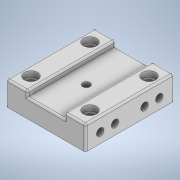
# Autodesk Inventor part: slidescentermount
Saved by Autodesk Inventor 2020 (Build 240168000, 168)
## iProperties
Created: 2019-12-20
Part Number: slidescentermount
Material: Generic
Document SubType Name: Modeling
Designer: xj82b
Density: 1 g/cm^3
Appearance: Default
Author: xj82b
Autodesk Inventor part; units mm, degrees
ref_plane "YZ Plane" through (0, 0, 0) normal (1, 0, 0) x (0, 1, 0)
ref_plane "XZ Plane" through (0, 0, 0) normal (0, 1, 0) x (-1, 0, 0)
ref_plane "XY Plane" through (0, 0, 0) normal (0, 0, 1) x (1, 0, 0)
sketch "Sketch1" plane through (0, 0, 0) normal (0, 1, 0) x (-1, 0, 0)
  line L0 (0, 0) -> (-43, 0)
  line L1 (-43, 0) -> (-43, -48)
  line L2 (-43, -48) -> (0, -48)
  line L3 (0, -48) -> (0, 0)
  circle A0 centre (-21.5, -22) radius 2
  point P0 (-43, -24)
  point P1 (-21.5, -48)
  dimension "d0" = 43
  dimension "d1" = 48
  dimension "d2" = 4
  dimension "d23" = 22
  constraints: 8 end point, 2 midpoint, 2 parallel, 1 centre point, 1 horizontal, 1 perpendicular, 1 vertical alignment
  measures "d0" distance of L2.end L1.end
  measures "d1" distance of L1.end L0.end
  measures "d2" diameter of A0
  measures "d23" distance from line of L0 A0.centre
extrude "Extrusion1" add sketch "Sketch1" along normal blind 13
sketch "Sketch2" plane through (0, 13, 0) normal (0, 1, 0) x (1, 0, 0)
  line L0 (11.5, 54.8346) -> (31.5, 54.8346)
  line L1 (31.5, 54.8346) -> (31.5, -5.4848)
  line L2 (31.5, -5.4848) -> (11.5, -5.4848)
  line L3 (11.5, -5.4848) -> (11.5, 54.8346)
  line L4 (43, 48) -> (0, 48) projected
  point P0 (0, 0)
  point P1 (21.5, 54.8346)
  point P2 (21.5, 48)
  dimension "d5" = 20
  constraints: 8 end point, 2 midpoint, 2 parallel, 1 horizontal, 1 perpendicular, 1 vertical alignment
  measures "d5" distance of L1.end L2.end
extrude "Extrusion2" cut sketch "Sketch2" against normal blind 3
sketch "Sketch3" plane through (0, 0, 0) normal (0, -1, 0) x (1, 0, 0)
  line L0 (23.5207, -18.5) -> (25.5415, -22)
  line L1 (25.5415, -22) -> (23.5207, -25.5)
  line L2 (23.5207, -25.5) -> (19.4793, -25.5)
  line L3 (19.4793, -25.5) -> (17.4585, -22)
  line L4 (17.4585, -22) -> (19.4793, -18.5)
  line L5 (19.4793, -18.5) -> (23.5207, -18.5)
  line L6 (43, -48) -> (0, -48) projected
  line L7 (0, -48) -> (0, 0) projected
  line L8 (0, 0) -> (43, 0) projected
  point P0 (21.5, -22)
  point P1 (21.5, -25.5)
  point P2 (21.5, -48)
  point P3 (0, -24)
  dimension "d8" = 7
  dimension "d24" = 22
  constraints: 12 end point, 3 midpoint, 1 parallel, 1 vertical alignment, 13 other
  measures "d8" distance between parallel lines of L4 L1
  measures "d24" distance from line of L8 point (21.5, -22)
extrude "Extrusion3" cut sketch "Sketch3" against normal blind 5
sketch "Sketch4" plane through (43, 0, 0) normal (1, 0, 0) x (0, 0, -1)
  circle A0 centre (24, 5.5) radius 2
  circle A1 centre (32, 5.5) radius 2
  circle A2 centre (16, 5.5) radius 2
  circle A3 centre (40, 5.5) radius 2
  circle A4 centre (8, 5.5) radius 2
  line L0 (0, 0) -> (48, 0) projected
  line L1 (0, 13) -> (48, 13) projected
  point P0 (24, 13)
  dimension "d11" = 4
  dimension "d12" = 4
  dimension "d13" = 4
  dimension "d14" = 4
  dimension "d15" = 4
  dimension "d16" = 8
  dimension "d17" = 8
  dimension "d18" = 8
  dimension "d19" = 8
  dimension "d20" = 5.5
  constraints: 5 centre point, 4 horizontal alignment, 1 midpoint, 1 vertical alignment
  measures "d11" diameter of A0
  measures "d12" diameter of A1
  measures "d13" diameter of A2
  measures "d14" diameter of A3
  measures "d15" diameter of A4
  measures "d16" distance of A1.centre A3.centre
  measures "d17" distance of A0.centre A1.centre
  measures "d18" distance of A0.centre A2.centre
  measures "d19" distance of A2.centre A4.centre
  measures "d20" distance from line of L0 A3.centre
extrude "Extrusion4" cut sketch "Sketch4" against normal through all contours A1 | A2 | A3 | A4
fillet "Fillet1" radius 1 7 edges at (11.5, 13, -24) (31.5, 13, -24) (11.5, 11.5, -48) (31.5, 11.5, -48) (37.25, 13, -48) (5.75, 13, -48) (21.5, 10, -48)
fillet "Fillet2" radius 1 15 edges at (43, 12.7071, -47.7071) (43, 6, -48) (43, 13, -23.5) (0, 12.7071, -47.7071) (0, 6, -48) (0, 13, -23.5) (11.2071, 12.7071, 0) (11.5, 11, 0) (5.25, 13, 0) (31.7929, 12.7071, 0) (31.5, 11, 0) (37.75, 13, 0) (0, 6.5, 0) (43, 6.5, 0) (21.5, 10, 0)
sketch "Sketch5" plane through (0, 13, 0) normal (0, 1, 0) x (1, 0, 0)
  circle A0 centre (5.5, 40) radius 2
  circle A1 centre (5.5, 8) radius 2
  line L0 (0, 47) -> (0, 1) projected
  line L1 (10.5, 48) -> (1, 48) projected
  circle A2 centre (37.5, 40) radius 2
  circle A3 centre (37.5, 8) radius 2
  line L2 (43, 1) -> (43, 47) projected
  point P0 (0, 0)
  dimension "d27" = 4
  dimension "d28" = 4
  dimension "d29" = 5.5
  dimension "d30" = 8
  dimension "d31" = 32
  dimension "d32" = 4
  dimension "d33" = 4
  dimension "d34" = 5.5
  constraints: 4 centre point, 2 horizontal alignment, 2 vertical alignment
  measures "d27" diameter of A0
  measures "d28" diameter of A1
  measures "d29" distance from line of L0 A0.centre
  measures "d30" distance from line of L1 A0.centre
  measures "d31" distance of A1.centre A0.centre
  measures "d32" diameter of A2
  measures "d33" diameter of A3
  measures "d34" distance from line of L2 A2.centre
extrude "Extrusion5" cut sketch "Sketch5" against normal through all
sketch "Sketch6" plane through (0, 13, 0) normal (0, 1, 0) x (1, 0, 0)
  circle A0 centre (5.5, 40) radius 3.6
  circle A1 centre (5.5, 8) radius 3.6
  circle A2 centre (37.5, 40) radius 3.6
  circle A3 centre (37.5, 8) radius 3.6
  circle A4 centre (37.5, 40) radius 2 projected
  circle A5 centre (37.5, 8) radius 2 projected
  circle A6 centre (5.5, 8) radius 2 projected
  circle A7 centre (5.5, 40) radius 2 projected
  point P0 (0, 0)
  dimension "d37" = 7.2
  dimension "d38" = 7.2
  dimension "d39" = 7.2
  dimension "d40" = 7.2
  constraints: 4 centre point, 4 concentric
  measures "d37" diameter of A0
  measures "d38" diameter of A1
  measures "d39" diameter of A2
  measures "d40" diameter of A3
extrude "Extrusion6" cut sketch "Sketch6" against normal blind 3
body "Solid1"
